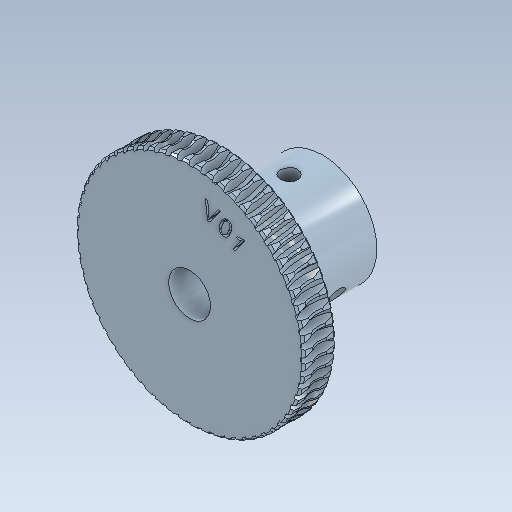
# Autodesk Inventor part: Worm Gear
Saved by Autodesk Inventor 2021.1 (Build 251245010, 245A)
## iProperties
CustomPartVersion: 1
Created: 2020-07-23
Part Number: Worm Gear
Material: Steel, Mild
Document SubType Name: Modeling
Designer: robst
Categories: <?xml version="1.0" encoding="UTF-16"?> <MemberInstance><Categories><FamilyTemplate><FamilyTemplateParameter ValueType="xs:double" Id="1" ObjectReferenceKey="da_z" ObjectType="kUserParameterObject"/><FamilyTemplateParameter ValueType="xs:double" Id="2" ObjectReferenceKey="da_b" ObjectType="kUserParameterObject"/><FamilyTemplateParameter ValueType="xs:double" Id="3" ObjectReferenceKey="da_beta" ObjectType="kUserParameterObject"/><FamilyTemplateParameter ValueType="xs:double" Id="4" ObjectReferenceKey="da_m" ObjectType="kUserParameterObject"/><FamilyTemplateParameter ValueType="xs:double" Id="5" ObjectReferenceKey="da_alpha" ObjectType="kUserParameterObject"/><FamilyTemplateParameter ValueType="xs:double" Id="6" ObjectReferenceKey="da_da" ObjectType="kUserParameterObject"/><FamilyTemplateParameter ValueType="xs:double" Id="7" ObjectReferenceKey="da_aw" ObjectType="kUserParameterObject"/><FamilyTemplateParameter ValueType="xs:double" Id="8" ObjectReferenceKey="da_px" ObjectType="kUserParameterObject"/><FamilyTemplateParameter ValueType="xs:double" Id="9" ObjectReferenceKey="da_d" ObjectType="kUserParameterObject"/><FamilyTemplateParameter ValueType="xs:double" Id="10" ObjectReferenceKey="da_dae" ObjectType="kUserParameterObject"/><FamilyTemplateParameter ValueType="xs:double" Id="11" ObjectReferenceKey="da_fi" ObjectType="kUserParameterObject"/><FamilyTemplateParameter ValueType="xs:string" Id="12" ObjectReferenceKey="EAIAABAAAAAWFwAAAAAAAIAAAAAAAAAA" ObjectType="83910656" SubObjectId="SurfaceGeometry"/></FamilyTemplate><ParamToTemplateMap><ParamToTemplate CategoryParameter="//CategoryParameter[@InternalName='046C89C9-8512-4d59-83FE-43B91F4F132A']" TemplateParameter="1"/><ParamToTemplate CategoryParameter="//CategoryParameter[@InternalName='2552DF32-E462-4b46-AEBF-C6C7768E72AC']" TemplateParameter="2"/><ParamToTemplate CategoryParameter="//CategoryParameter[@InternalName='C9EE641D-15FC-4fae-A226-E94C4372FDD7']" TemplateParameter="3"/><ParamToTemplate><ParamToTemplate CategoryParameter="//CategoryParameter[@InternalName='00B6519A-459B-49c7-AD84-2E56D39A5744']" ConstantValue="0.000000"/></ParamToTemplate><ParamToTemplate><ParamToTemplate CategoryParameter="//CategoryParameter[@InternalName='04B31F0E-C7A6-4894-AA32-9629BEFACF47']" ConstantValue="1.000000"/></ParamToTemplate><ParamToTemplate><ParamToTemplate CategoryParameter="//CategoryParameter[@InternalName='43CBEC2E-7847-49e7-A936-2F7889FCB2D9']" ConstantValue="0.200000"/></ParamToTemplate><ParamToTemplate><ParamToTemplate CategoryParameter="//CategoryParameter[@InternalName='B1EFC894-105D-4ebd-86BF-FA20ED196853']" ConstantValue="0.300000"/></ParamToTemplate><ParamToTemplate><ParamToTemplate CategoryParameter="//CategoryParameter[@InternalName='51175063-3D10-4879-93E8-6246FE8B403D']" ConstantValue="2061532430.657340"/></ParamToTemplate><ParamToTemplate><ParamToTemplate CategoryParameter="//CategoryParameter[@InternalName='A3A52E27-4454-46a9-B0BD-C932399B70AF']" ConstantValue="0.300000"/></ParamToTemplate><ParamToTemplate CategoryParameter="//CategoryParameter[@InternalName='91B76062-C214-41d9-B1B9-14D2AB99603D']" TemplateParameter="4"/><ParamToTemplate CategoryParameter="//CategoryParameter[@InternalName='2D373A89-B862-43d6-8D0B-0CBF12AB9F6C']" TemplateParameter="5"/><ParamToTemplate CategoryParameter="//CategoryParameter[@InternalName='37777632-D6A2-4fac-9D53-DB8ACD95C989']" TemplateParameter="6"/><ParamToTemplate CategoryParameter="//CategoryParameter[@InternalName='FD1017F1-B727-4f7e-9707-0F86F1FF9423']" TemplateParameter="7"/><ParamToTemplate CategoryParameter="//CategoryParameter[@InternalName='3BF567DA-17EF-48d8-80EA-D119B07F6463']" TemplateParameter="8"/><ParamToTemplate CategoryParameter="//CategoryParameter[@InternalName='BF5A1E7E-5373-4a22-AAD3-F583781FCF3C']" TemplateParameter="9"/><ParamToTemplate CategoryParameter="//CategoryParameter[@InternalName='2A200944-5A8C-41ca-B96E-8520D2E510F1']" TemplateParameter="10"/><ParamToTemplate CategoryParameter="//CategoryParameter[@InternalName='E77AC4FD-7B43-4566-B0ED-7CA70B976BC8']" TemplateParameter="11"/><ParamToTemplate><ParamToTemplate CategoryParameter="//CategoryParameter[@InternalName='D4F72237-D604-435a-AD0B-F738B7463A00']" ConstantValue="110.000000"/></ParamToTemplate><ParamToTemplate><ParamToTemplate CategoryParameter="//CategoryParameter[@InternalName='9E1B4470-B2D3-4ff1-B813-535BB4CDF51A']" ConstantValue="1999479.615019"/></ParamToTemplate><ParamToTemplate><ParamToTemplate CategoryParameter="//CategoryParameter[@InternalName='A7A89E9A-52E6-4d4f-86CF-A81914F22AA4']" ConstantValue="250000000.000000"/></ParamToTemplate><ParamToTemplate><ParamToTemplate CategoryParameter="//CategoryParameter[@InternalName='B02FABAC-469F-4ad8-A219-DB4578299DF6']" ConstantValue="250000000.000000"/></ParamToTemplate><ParamToTemplate><ParamToTemplate CategoryParameter="//CategoryParameter[@InternalName='E6981962-40D5-4343-A0AD-C263FCC47E10']" ConstantValue="9.000000"/></ParamToTemplate><ParamToTemplate><ParamToTemplate CategoryParameter="//CategoryParameter[@InternalName='B958E99F-2BCD-4955-8634-793EB7B37B89']" ConstantValue="8.000000"/></ParamToTemplate><ParamToTemplate><ParamToTemplate CategoryParameter="//CategoryParameter[@InternalName='4AD49A87-569D-440f-A541-E3B52A6A9DCE']" ConstantValue="1219.200000"/></ParamToTemplate><ParamToTemplate><ParamToTemplate CategoryParameter="//CategoryParameter[@InternalName='4E5813A0-330D-4b41-BE23-D880B01A1D55']" ConstantValue="1654741.750360"/></ParamToTemplate><ParamToTemplate><ParamToTemplate CategoryParameter="//CategoryParameter[@InternalName='19EB8C86-AA88-4253-B4AA-2F5DF1CE171A']" ConstantValue="5515.805835"/></ParamToTemplate><ParamToTemplate CategoryParameter="//CategoryParameter[@InternalName='27C3BAF2-7550-4e4b-AE2C-0DB134B7D9B7']" TemplateParameter="12"/></ParamToTemplateMap><Category DisplayName="Gear" InternalName="DC85795E-93AB-48d5-8EEE-5A27447B64BD" Mnemonic="Gear"><CategoryParameter DisplayName="z" InternalName="046C89C9-8512-4d59-83FE-43B91F4F132A" Mnemonic="z"/><CategoryParameter DisplayName="b|.2|" InternalName="2552DF32-E462-4b46-AEBF-C6C7768E72AC" Mnemonic="b"/><CategoryParameter DisplayName="||b|" InternalName="C9EE641D-15FC-4fae-A226-E94C4372FDD7" Mnemonic="beta"/><CategoryParameter DisplayName="x" InternalName="00B6519A-459B-49c7-AD84-2E56D39A5744" Mnemonic="x"/><CategoryParameter DisplayName="a*" InternalName="04B31F0E-C7A6-4894-AA32-9629BEFACF47" Mnemonic="a"/><CategoryParameter DisplayName="c*" InternalName="43CBEC2E-7847-49e7-A936-2F7889FCB2D9" Mnemonic="c"/><CategoryParameter DisplayName="r|.f|*" InternalName="B1EFC894-105D-4ebd-86BF-FA20ED196853" Mnemonic="rf"/><CategoryParameter DisplayName="E" InternalName="51175063-3D10-4879-93E8-6246FE8B403D" Mnemonic="E"/><CategoryParameter DisplayName="||m|" InternalName="A3A52E27-4454-46a9-B0BD-C932399B70AF" Mnemonic="mi"/><Category DisplayName="WormGear" InternalName="1B25C7EF-093B-4025-B3D3-619CD2A4550C" Mnemonic="WormGear"><CategoryParameter DisplayName="m" InternalName="91B76062-C214-41d9-B1B9-14D2AB99603D" Mnemonic="m"/><CategoryParameter DisplayName="||a|" InternalName="2D373A89-B862-43d6-8D0B-0CBF12AB9F6C" Mnemonic="alpha"/><CategoryParameter DisplayName="d|.a|" InternalName="37777632-D6A2-4fac-9D53-DB8ACD95C989" Mnemonic="da"/><CategoryParameter DisplayName="a|.w|" InternalName="FD1017F1-B727-4f7e-9707-0F86F1FF9423" Mnemonic="aw"/><CategoryParameter DisplayName="p|.x|" InternalName="3BF567DA-17EF-48d8-80EA-D119B07F6463" Mnemonic="px"/><CategoryParameter DisplayName="d" InternalName="BF5A1E7E-5373-4a22-AAD3-F583781FCF3C" Mnemonic="d"/><CategoryParameter DisplayName="dae" InternalName="2A200944-5A8C-41ca-B96E-8520D2E510F1" Mnemonic="dae"/><CategoryParameter DisplayName="||d|" InternalName="E77AC4FD-7B43-4566-B0ED-7CA70B976BC8" Mnemonic="fi"/><CategoryParameter DisplayName="VHV" InternalName="D4F72237-D604-435a-AD0B-F738B7463A00" Mnemonic="VHV"/><CategoryParameter DisplayName="||s||.Hlim|" InternalName="9E1B4470-B2D3-4ff1-B813-535BB4CDF51A" Mnemonic="sHlim"/><CategoryParameter DisplayName="N|.Flim|" InternalName="A7A89E9A-52E6-4d4f-86CF-A81914F22AA4" Mnemonic="NFlim"/><CategoryParameter DisplayName="N|.Hlim|" InternalName="B02FABAC-469F-4ad8-A219-DB4578299DF6" Mnemonic="NHlim"/><CategoryParameter DisplayName="q|.F|" InternalName="E6981962-40D5-4343-A0AD-C263FCC47E10" Mnemonic="qF"/><CategoryParameter DisplayName="q|.H|" InternalName="B958E99F-2BCD-4955-8634-793EB7B37B89" Mnemonic="qH"/><CategoryParameter DisplayName="v|.max|" InternalName="4AD49A87-569D-440f-A541-E3B52A6A9DCE" Mnemonic="maxv"/><CategoryParameter DisplayName="S|.n|" InternalName="4E5813A0-330D-4b41-BE23-D880B01A1D55" Mnemonic="Sn"/><CategoryParameter DisplayName="K|.w|" InternalName="19EB8C86-AA88-4253-B4AA-2F5DF1CE171A" Mnemonic="Kw"/><CategoryParameter DisplayName="PitchDiameter" InternalName="27C3BAF2-7550-4e4b-AE2C-0DB134B7D9B7" Mnemonic="IDS_PITCHDIAM"/></Category></Category></Categories></MemberInstance>
Density: 7.86 g/cm^3
Appearance: Steel Blue
Author: robst
Autodesk Inventor part; units mm, degrees
ref_plane "Tooth Plane" through (0, -10, 0) normal (-0.0995037, 0, 0.9950372) x (0, 1, 0)
sketch "Base Body Sketch" plane through (0, 0, 0) normal (1, 0, 0) x (0, 1, 0)
  line L0 (0, -8.61) -> (0, 8.61) projected
  line L1 (0, 6.15) -> (42.6119, 6.15)
  line L2 (42.6119, 6.15) -> (43.2956, 5.3848)
  line L3 (-10.0902, 0) -> (60.541, 0) construction
  circle A0 centre (48.1062, 0) radius 5.4978
  line L4 (43.2956, 5.3848) -> (43.2956, -5.3848)
  line L5 (0, -6.15) -> (42.6119, -6.15)
  line L6 (0, 6.15) -> (0, -6.15)
  line L7 (42.6119, -6.15) -> (43.2956, -5.3848)
  dimension "d50" = 48.223
  dimension "d87" = 86.5911
  dimension "d89" = 10.9957
  dimension "d92" = 12.3
  dimension "d93" = 48.1062
  constraints: 14 end point, 3 symmetric about line, 2 perpendicular, 2 point on line, 1 centre point, 1 collinear
  measures "d50" angle of L2 L1
  measures "d87" diameter of L4 L0
  measures "d89" diameter of A0
  measures "d92" distance of L1.start L5.start
  measures "d93" distance from line of A0.centre L6
revolve "Base Body" add sketch "Base Body Sketch" angle 360 about axis through (0, 0, 0) along (0, 0, 1) picked at (43.1501, -0.5472) contours L0 L1 L2 L4 A0 L7 L5 | A0 L4
revolve "Base Body2" cut sketch "Base Body Sketch" angle 360 about axis through (0, 0, 0) along (0, 0, 1) contours L4 A0 | A0 L4
sketch "Tooth Sketch" plane through (0, -10, 0) normal (-0.0995037, 0, 0.9950372) x (0, 1, 0)
  line L0 (10, 2.4979) -> (10, -2.4979) projected
  line L1 (-36.8805, 0) -> (-25.6519, 0) projected
  line L2 (-38.1062, 1.8957) -> (-38.1062, -1.8957)
  line L3 (-38.1062, -1.8957) -> (-32.8832, -1.8957)
  line L4 (-32.8832, -1.8957) -> (-29.5845, -0.6951)
  line L5 (-29.5845, -0.6951) -> (-29.5845, 0)
  line L6 (-29.5845, 0.6951) -> (-32.8832, 1.8957)
  line L7 (-32.8832, 1.8957) -> (-38.1062, 1.8957)
  line L8 (-29.5845, 0.6951) -> (-29.5845, 0)
  line L9 (-31.2339, 0) -> (-31.2339, -1.2954) construction
  dimension "d38" = 48.1062
  dimension "d39" = 20
  dimension "d40" = 5.223
  dimension "d41" = 6.8723
  dimension "d42" = 1.2954
  constraints: 16 end point, 4 perpendicular, 3 equal length, 2 point on line, 1 midpoint, 1 parallel, 1 vertical
  measures "d38" distance between parallel lines of L0 L2
  measures "d39" angle of L6 L7
  measures "d40" distance of L6.end L2.start
  measures "d41" distance between parallel lines of L2 L9
  measures "d42" distance of L9.start L9.end
sketch "Sketch8" plane through (0, 0, 6.15) normal (0, 0, 1) x (1, 0, 0)
  circle A0 centre (0, 0) radius 42.6119 projected
  circle A1 centre (0, 0) radius 41.2339
  dimension "d77" = 82.4677
  constraints: 1 centre point, 1 coincident
  measures "d77" diameter of A1
surface extrude "Pitch Diameter" sketch "Sketch8" against normal blind 12.3 shown no curves A1
ref_plane "Work Plane13" through (0, 0, 0) normal (-0.052336, 0.9986295, 0) x (0, 0, 1)
revolve "Tooth" cut sketch "Tooth Sketch" angle 360 about axis through (-1.8863, -48.1062, -0.1886) along (0.9950372, 0, 0.0995037)
pattern_circular "Tooth Pattern" count 60 over 360 about axis through (0, 0, 0) along (0, 0, 1) of "Tooth"
ref_plane "Work Plane14" through (0, 0, 0) normal (0.9986295, 0.052336, 0) x (0, 0, 1)
ref_plane "Work Plane15" through (0, 0, 0) normal (0, -1, 0) x (0, 0, 1)
sketch "Sketch9" plane through (61.5, -48.1062, 6.15) normal (0, 0, 1) x (1, 0, 0)
  circle A0 centre (-61.5, 48.1062) radius 7.9375
  dimension "d94" = 15.875
  constraints: 1 centre point, 1 coincident
  measures "d94" diameter of A0
extrude "Extrusion1" cut sketch "Sketch9" against normal through all
sketch "Sketch11" plane through (-61.5, -48.1062, -6.15) normal (0, 0, -1) x (-1, 0, 0)
  circle A0 centre (-61.5, 48.1062) radius 7.9375 projected
  circle A1 centre (-61.5, 48.1062) radius 20.6375
  circle A2 centre (-61.5, 48.1062) radius 7.9375
  dimension "d100" = 41.275
  constraints: 2 centre point, 2 coincident, 1 concentric
  measures "d100" diameter of A1
extrude "Extrusion3" add sketch "Sketch11" along normal blind 38.1
ref_plane "Work Plane16" through (0, 20.6375, -6.15) normal (0, 1, 0) x (-1, 0, 0)
sketch "Sketch12" plane through (0, 20.6375, -6.15) normal (0, 1, 0) x (-1, 0, 0)
  line L0 (-20.6375, 0) -> (-20.6375, -38.1) projected
  line L1 (20.6375, 0) -> (20.6375, -38.1) projected
  line L2 (-20.6375, -38.1) -> (20.6375, -38.1) projected
  line L3 (1.3136, 0) -> (-0.0836, 0) projected
  point P0 (0, 6.15)
  point P1 (0, -25.4)
  dimension "d116" = 25.4
  measures "d116" distance from line of L3 point (0, -25.4)
hole "Hole3" at (0, 20.6375, -31.55) direction (0, -1, 0) diameter 5.1054 depth 15.24 tip angle 118 counterbore diameter 6.5278 counterbore depth 9.525 clearance for "Hex Machine Screw" size "#10" standard "Ansi Unified Screw Threads"
pattern_circular "Circular Pattern2" count 3 over 360 about axis through (0, 0, 0) along (0, 0, 1) of "Hole3"
sketch "Sketch13" plane through (61.5, -48.1062, 6.15) normal (0, 0, 1) x (1, 0, 0)
  circle A0 centre (-61.5, 48.1062) radius 31.75 construction
  line L0 (-54.7274, 75.8709) -> (-55.4961, 82.635)
  line L1 (-55.4961, 82.635) -> (-54.6158, 82.405)
  line L2 (-54.6158, 82.405) -> (-54.1851, 77.5251)
  spline S0 degree 2 poles (-54.1851, 77.5251) (-54.1326, 76.9411) (-54.1239, 76.4386) knots 0 0 0 1 1 1
  spline S1 degree 2 poles (-54.1239, 76.4386) (-53.8525, 76.9029) (-53.5342, 77.355) knots 0 0 0 1 1 1
  line L3 (-53.5342, 77.355) -> (-50.7057, 81.3832)
  line L4 (-50.7057, 81.3832) -> (-49.8769, 81.1666)
  line L5 (-49.8769, 81.1666) -> (-53.8892, 75.6519)
  line L6 (-53.8892, 75.6519) -> (-54.7274, 75.8709)
  spline S2 degree 2 poles (-49.7488, 77.6292) (-49.2635, 78.6472) (-48.2526, 79.6879) (-47.1125, 79.9648) (-46.4834, 79.6648) knots 0 0 0 1 2 3 3 3
  spline S3 degree 2 poles (-46.4834, 79.6648) (-46.0247, 79.4461) (-45.5027, 78.7415) (-45.386, 77.828) (-45.6073, 76.7003) (-46.0135, 75.8483) knots 0 0 0 1 2 3 4 4 4
  spline S4 degree 2 poles (-46.0135, 75.8483) (-46.4946, 74.8391) (-47.5012, 73.7963) (-48.6477, 73.5171) (-49.2724, 73.815) knots 0 0 0 1 2 3 3 3
  spline S5 degree 2 poles (-49.2724, 73.815) (-50.1025, 74.2107) (-50.2931, 75.0255) knots 0 0 0 1 1 1
  spline S6 degree 2 poles (-50.2931, 75.0255) (-50.5174, 76.0171) (-49.7488, 77.6292) knots 0 0 0 1 1 1
  spline S7 degree 2 poles (-49.0236, 77.2835) (-49.6985, 75.868) (-49.4824, 74.6229) (-48.9975, 74.3917) knots 0 0 0 1 2 2 2
  spline S8 degree 2 poles (-48.9975, 74.3917) (-48.5169, 74.1626) (-47.4115, 74.783) (-46.7387, 76.1941) knots 0 0 0 1 2 2 2
  spline S9 degree 2 poles (-46.7387, 76.1941) (-46.0638, 77.6096) (-46.2799, 78.8547) (-46.7692, 79.088) knots 0 0 0 1 2 2 2
  spline S10 degree 2 poles (-46.7692, 79.088) (-47.2541, 79.3192) (-47.7383, 79.046) knots 0 0 0 1 1 1
  spline S11 degree 2 poles (-47.7383, 79.046) (-48.3508, 78.6946) (-49.0236, 77.2835) knots 0 0 0 1 1 1
  line L7 (-44.2845, 70.9284) -> (-44.9201, 71.3793)
  line L8 (-44.9201, 71.3793) -> (-42.0467, 75.4293)
  spline S12 degree 2 poles (-42.0467, 75.4293) (-42.4297, 75.3747) (-43.4866, 75.4658) (-43.8611, 75.5653) knots 0 0 0 1 2 2 2
  line L9 (-43.8611, 75.5653) -> (-43.4242, 76.1811)
  spline S13 degree 2 poles (-43.4242, 76.1811) (-42.7148, 76.0517) (-41.4106, 76.2005) (-41.0067, 76.4184) knots 0 0 0 1 2 2 2
  line L10 (-41.0067, 76.4184) -> (-40.5962, 76.1271)
  line L11 (-40.5962, 76.1271) -> (-44.2845, 70.9284)
  dimension "d113" = 63.5
  constraints: 1 centre point, 1 coincident, 1 other
  measures "d113" diameter of A0
extrude "Extrusion4" cut sketch "Sketch13" against normal blind 2.54
equation "\"d50\" = da_fi"
equation "\"d87\" = da_dae"
equation "\"d89\" = 2 * da_aw - da_da"
equation "\"d92\" = da_b"
equation "\"d93\" = da_aw"
equation "\"d94\" = aRsCenterHole"
equation "\"d100\" = aRsOuterPostDiameter"
equation "\"d38\" = da_aw"
equation "\"d39\" = da_alfat"
equation "\"d40\" = 0.5 * da_df1"
equation "\"d41\" = 0.5 * da_d1"
equation "\"d42\" = 0.3 * da_px"
equation "\"d77\" = da_dw"
equation "\"d78\" = da_b"
equation "\"da_aw\" = 48.10617"
equation "\"da_fi\" = 48.2232deg"
equation "\"da_b\" = 12.3"
equation "\"da_df\" = 79.16902"
equation "\"da_da\" = 85.21665"
equation "\"da_beta\" = 5.710593deg"
equation "\"da_alfat\" = 20deg"
equation "\"da_df1\" = 10.44591"
equation "\"da_da1\" = 16.49355"
equation "\"da_d1\" = 13.74462"
equation "\"da_px\" = 4.318"
equation "\"d68\" = da_aw"
equation "\"da_dw\" = 82.46773"
equation "\"da_rightdir\" = 0"
equation "\"d86\" = da_aw"
equation "\"da_dae\" = 86.59111"
equation "\"aRsCenterHole\" = 15.875"
equation "\"aRsOuterPostDiameter\" = 41.275"
body "Solid1"
body "Srf1"
